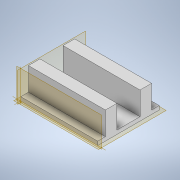
# Autodesk Inventor part: Shoket2.0
Saved by Autodesk Inventor 2022 (Build 260153000, 153)
## iProperties
Created: 2022-05-12
Part Number: Shoket2.0
Material: Generic
Document SubType Name: Modeling
Designer: dovalle
Density: 1 g/cm^3
Appearance: Default
Author: dovalle
Autodesk Inventor part; units mm, degrees
sketch "Sketch1" plane through (0, 0, 0) normal (1, 0, 0) x (0, 1, 0)
  line L0 (0, 0) -> (1, 0)
  line L1 (1, 0) -> (1, -2)
  line L2 (1, -2) -> (7, -2)
  line L3 (7, -2) -> (7, -5)
  line L4 (7, -5) -> (1, -5)
  line L5 (1, -5) -> (1, -11)
  line L6 (1, -11) -> (7, -11)
  line L7 (7, -11) -> (7, -14)
  line L8 (7, -14) -> (1, -14)
  line L9 (1, -14) -> (1, -16)
  line L10 (1, -16) -> (0, -16)
  line L11 (0, -16) -> (0, 0)
  constraints: 24 end point, 6 perpendicular, 3 point on line, 1 horizontal, 1 vertical
extrude "Extrusion1" add sketch "Sketch1" along normal blind 20
body "Solid1"
